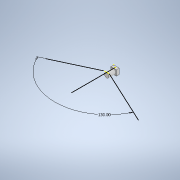
# Autodesk Inventor part: HDzero runcam nano spacer
Saved by Autodesk Inventor 2020 (Build 240168000, 168)
## iProperties
Created: 2022-05-06
Part Number: HDzero runcam nano spacer
Material: Generic
Document SubType Name: Modeling
Designer: Steven
Density: 1 g/cm^3
Appearance: Default
Author: Steven
Autodesk Inventor part; units mm, degrees
ref_plane "YZ Plane" through (0, 0, 0) normal (1, 0, 0) x (0, 1, 0)
ref_plane "XZ Plane" through (0, 0, 0) normal (0, 1, 0) x (-1, 0, 0)
ref_plane "XY Plane" through (0, 0, 0) normal (0, 0, 1) x (1, 0, 0)
sketch "Sketch1" plane through (0, 0, 0) normal (0, 0, 1) x (1, 0, 0)
  line L0 (0, 0) -> (14.45, 0)
  line L1 (14.45, 0) -> (14.45, 14.45)
  line L2 (14.45, 14.45) -> (0, 14.45)
  line L3 (0, 14.45) -> (0, 0)
  dimension "d0" = 14.45
  dimension "d1" = 14.45
  constraints: 8 end point, 2 parallel, 1 horizontal, 1 perpendicular
  measures "d0" distance of L2.end L1.end
  measures "d1" distance of L1.end L0.end
extrude "Extrusion1" add sketch "Sketch1" along normal blind 7.5
sketch "Sketch6" plane through (0, 0, 7.5) normal (0, 0, 1) x (1, 0, 0)
  line L0 (14.45, 0) -> (14.45, 14.45) construction
  line L1 (14.45, 7.225) -> (0, 7.225) construction
  line L2 (0, 14.45) -> (0, 0) construction
  circle A0 centre (7.225, 7.225) radius 6
  dimension "d14" = 12
  constraints: 3 midpoint, 2 end point, 1 centre point
  measures "d14" diameter of A0
sketch "Sketch7" plane through (0, 0, 0) normal (-1, 0, 0) x (0, 0, 1)
  line L0 (0, 14.45) -> (0, 0) projected
  line L1 (0, 0) -> (7.5, 0) projected
  line L2 (7.5, 14.45) -> (7.5, 0) projected
  line L3 (0, 14.45) -> (7.5, 14.45) projected
  dimension "d15" = 7.5
  measures "d15" distance of L0.start L2.start
extrude "Extrusion4" add sketch "Sketch6" along normal blind 18
sketch "Sketch8" plane through (0, 14.45, 0) normal (0, 1, 0) x (1, 0, 0)
  line L0 (14.45, 0) -> (0, 0) projected
  line L1 (0, 0) -> (14.45, 0) construction
  line L2 (7.225, 0) -> (7.225, -5) construction
  line L3 (7.225, -5) -> (9.4124, -5) construction
  circle A0 centre (7.225, -4) radius 1
  dimension "d18" = 5
  dimension "d19" = 2
  constraints: 4 end point, 1 centre point, 1 horizontal, 1 midpoint, 1 point on line, 1 tangent, 1 vertical
  measures "d18" distance of L2.start L2.end
  measures "d19" diameter of A0
extrude "Extrusion5" cut sketch "Sketch8" against normal up to surface (14.45 mm away)
sketch "Sketch10" plane through (0, 14.45, 0) normal (0, 1, 0) x (1, 0, 0)
  circle A0 centre (7.225, -4) radius 1 projected
  line L0 (7.225, -4) -> (7.225, -117.6084)
  line L1 (-0.5469, -26.3262) -> (-104.2988, -74.7065)
  line L2 (1.225, -25.5) -> (13.225, -25.5) projected
  line L3 (13.225, -25.5) -> (157.0278, -92.5563)
  point P0 (0, 0)
  dimension "d22" = 130
  constraints: 6 end point, 1 point on line, 1 vertical, 1 other
  measures "d22" angle of L3 L1
body "Solid1"
